Autodesk Fusion 360 part; units mm, degrees
note: some values were not read from the file. Set by a fixed rule: which sketch regions a step uses.
(part 2 of 2)
  line L440 (18.6477, 82.7525) -> (18.6477, 82.7527)
  line L441 (18.6477, 82.7527) -> (18.6477, 82.7525)
  circle A451 centre (18.1478, 85.2926) radius 0.754
  arc A452 (17.648, 85.2925) -> (18.6477, 85.2925) centre (18.1478, 85.2925) ccw
  arc A453 (18.6477, 85.2927) -> (17.648, 85.2927) centre (18.1478, 85.2927) ccw
  line L442 (17.648, 85.2927) -> (17.648, 85.2925)
  line L443 (17.648, 85.2925) -> (17.648, 85.2927)
  line L444 (18.6477, 85.2925) -> (18.6477, 85.2927)
  line L445 (18.6477, 85.2927) -> (18.6477, 85.2925)
  arc A454 (78.2438, 58.2496) -> (78.2438, 59.2496) centre (78.2438, 58.7496) ccw
  arc A455 (78.1938, 59.2496) -> (78.1938, 58.2496) centre (78.1938, 58.7496) ccw
  line L446 (78.2438, 58.2496) -> (78.1938, 58.2496)
  line L447 (78.1938, 58.2496) -> (78.2438, 58.2496)
  line L448 (78.2438, 59.2496) -> (78.1938, 59.2496)
  line L449 (78.1938, 59.2496) -> (78.2438, 59.2496)
  arc A456 (78.2438, 55.7096) -> (78.2438, 56.7096) centre (78.2438, 56.2096) ccw
  arc A457 (78.1938, 56.7096) -> (78.1938, 55.7096) centre (78.1938, 56.2096) ccw
  line L450 (78.2438, 55.7096) -> (78.1938, 55.7096)
  line L451 (78.1938, 55.7096) -> (78.2438, 55.7096)
  line L452 (78.2438, 56.7096) -> (78.1938, 56.7096)
  line L453 (78.1938, 56.7096) -> (78.2438, 56.7096)
  arc A458 (78.2438, 53.1696) -> (78.2438, 54.1696) centre (78.2438, 53.6696) ccw
  arc A459 (78.1938, 54.1696) -> (78.1938, 53.1696) centre (78.1938, 53.6696) ccw
  line L454 (78.2438, 53.1696) -> (78.1938, 53.1696)
  line L455 (78.1938, 53.1696) -> (78.2438, 53.1696)
  line L456 (78.2438, 54.1696) -> (78.1938, 54.1696)
  line L457 (78.1938, 54.1696) -> (78.2438, 54.1696)
  arc A460 (78.2438, 60.7896) -> (78.2438, 61.7896) centre (78.2438, 61.2896) ccw
  arc A461 (78.1938, 61.7896) -> (78.1938, 60.7896) centre (78.1938, 61.2896) ccw
  line L458 (78.2438, 60.7896) -> (78.1938, 60.7896)
  line L459 (78.1938, 60.7896) -> (78.2438, 60.7896)
  line L460 (78.1938, 61.7896) -> (78.2438, 61.7896)
  line L461 (78.2438, 61.7896) -> (78.1938, 61.7896)
  arc A462 (81.4368, 16.5156) -> (81.4368, 17.7156) centre (81.4368, 17.1156) ccw
  arc A463 (83.6368, 17.7156) -> (83.6368, 16.5156) centre (83.6368, 17.1156) ccw
  line L462 (83.6368, 16.5156) -> (81.4368, 16.5156)
  line L463 (81.4368, 16.5156) -> (83.6368, 16.5156)
  line L464 (81.4368, 17.7156) -> (83.6368, 17.7156)
  line L465 (83.6368, 17.7156) -> (81.4368, 17.7156)
  arc A464 (87.6368, 13.0156) -> (86.4368, 13.0156) centre (87.0368, 13.0156) ccw
  arc A465 (86.4368, 15.2156) -> (87.6368, 15.2156) centre (87.0368, 15.2156) ccw
  line L466 (86.4368, 15.2156) -> (86.4368, 13.0156)
  line L467 (86.4368, 13.0156) -> (86.4368, 15.2156)
  line L468 (87.6368, 13.0156) -> (87.6368, 15.2156)
  line L469 (87.6368, 15.2156) -> (87.6368, 13.0156)
  arc A466 (81.4368, 9.9156) -> (81.4368, 11.1156) centre (81.4368, 10.5156) ccw
  arc A467 (83.6368, 11.1156) -> (83.6368, 9.9156) centre (83.6368, 10.5156) ccw
  line L470 (81.4368, 9.9156) -> (83.6368, 9.9156)
  line L471 (83.6368, 9.9156) -> (81.4368, 9.9156)
  line L472 (83.6368, 11.1156) -> (81.4368, 11.1156)
  line L473 (81.4368, 11.1156) -> (83.6368, 11.1156)
  circle A468 centre (83.9338, 61.6706) radius 0.4445
  circle A469 centre (83.9338, 59.1306) radius 0.4445
  circle A470 centre (83.9338, 59.1306) radius 0.7874
  circle A471 centre (83.9338, 56.5906) radius 0.4445
  circle A472 centre (83.9338, 56.5906) radius 0.7874
  circle A473 centre (83.9338, 54.0506) radius 0.4445
  circle A474 centre (83.9338, 54.0506) radius 0.7874
  circle A475 centre (38.3408, 61.2198) radius 1.016
  circle A476 centre (5.3208, 60.9658) radius 1.016
  circle A477 centre (5.3208, 16.0078) radius 1.016
  circle A478 centre (38.3408, 16.0078) radius 1.016
  circle A479 centre (50.5049, 4.6197) radius 1.016
  circle A480 centre (72.4048, 4.6197) radius 1.016
  circle A481 centre (50.5049, 61.1197) radius 1.016
  circle A482 centre (72.4048, 61.1197) radius 1.016
  circle A483 centre (71.3075, 67.3056) radius 1.5
  circle A484 centre (50.9806, 67.3056) radius 1.5
  circle A485 centre (50.9806, 97.8054) radius 1.5
  circle A486 centre (71.3075, 97.8456) radius 1.5
  circle A487 centre (95.8825, 46.7984) radius 1.4999
  circle A488 centre (95.8543, 38.3133) radius 1.4999
  circle A489 centre (19.2908, 71.0686) radius 1
  circle A490 centre (19.2908, 91.8966) radius 1
  circle A491 centre (42.4048, 91.8966) radius 1
  circle A492 centre (42.4048, 71.0686) radius 1
  circle A493 centre (82.5368, 6.5155) radius 1.25
  arc A494 (104.4344, 98.5006) -> (97.6244, 105.3106) centre (97.6244, 98.5006) ccw
  line L474 (3.6444, 105.3106) -> (97.6244, 105.3106)
  arc A495 (3.6444, 105.3106) -> (-3.1656, 98.5006) centre (3.6444, 98.5006) ccw
  line L475 (-3.1656, -5.4794) -> (-3.1656, 98.5006)
  line L476 (104.4344, 98.5006) -> (104.4344, 4.5206)
  line L477 (-3.1656, -5.4794) -> (-3.1656, -49.4794)
  line L478 (104.4344, 4.5206) -> (104.4344, -49.4794)
  line L479 (2.8344, -55.4794) -> (98.4344, -55.4794)
  arc A496 (-3.1656, -49.4794) -> (2.8344, -55.4794) centre (2.8344, -49.4794) ccw
  arc A497 (98.4344, -55.4794) -> (104.4344, -49.4794) centre (98.4344, -49.4794) ccw
  arc A498 (108.4344, 98.5006) -> (97.6244, 109.3106) centre (97.6244, 98.5006) ccw
  line L480 (3.6444, 109.3106) -> (97.6244, 109.3106)
  arc A499 (3.6444, 109.3106) -> (-7.1656, 98.5006) centre (3.6444, 98.5006) ccw
  line L481 (-7.1656, -5.4794) -> (-7.1656, 98.5006)
  line L482 (-7.1656, -5.4794) -> (-7.1656, -49.4794)
  arc A500 (-7.1656, -49.4794) -> (2.8344, -59.4794) centre (2.8344, -49.4794) ccw
  line L483 (2.8344, -59.4794) -> (98.4344, -59.4794)
  arc A501 (98.4344, -59.4794) -> (108.4344, -49.4794) centre (98.4344, -49.4794) ccw
  line L484 (108.4344, 4.5206) -> (108.4344, -49.4794)
  line L485 (108.4344, 98.5006) -> (108.4344, 4.5206)
  arc A502 (105.9344, 98.5006) -> (97.6244, 106.8106) centre (97.6244, 98.5006) ccw
  line L486 (3.6444, 106.8106) -> (97.6244, 106.8106)
  arc A503 (3.6444, 106.8106) -> (-4.6656, 98.5006) centre (3.6444, 98.5006) ccw
  line L487 (-4.6656, -5.4794) -> (-4.6656, 98.5006)
  line L488 (-4.6656, -5.4794) -> (-4.6656, -49.4794)
  arc A504 (-4.6656, -49.4794) -> (2.8344, -56.9794) centre (2.8344, -49.4794) ccw
  line L489 (2.8344, -56.9794) -> (98.4344, -56.9794)
  arc A505 (98.4344, -56.9794) -> (105.9344, -49.4794) centre (98.4344, -49.4794) ccw
  line L490 (105.9344, 4.5206) -> (105.9344, -49.4794)
  line L491 (105.9344, 98.5006) -> (105.9344, 4.5206)
  point P0 (-3.1656, -55.4794)
  point P1 (104.4344, -55.4794)
  dimension "d2" = 50
  dimension "d3" = 60
  dimension "d4" = 6
  dimension "d5" = 6
  dimension "d6" = 56.19
  dimension "d7" = 101.6
  dimension "d8" = -4
  dimension "d13" = 101.6
  dimension "d14" = -1.5
  constraint concentric A0 A494
  constraint concentric A3 A495
  constraint tangent A495 L475
  constraint tangent L474 A495
  constraint tangent A494 L474
  constraint tangent A494 L476
  constraint vertical L477
  constraint parallel L475 L477
  constraint vertical L478
  constraint parallel L476 L478
  constraint perpendicular L478 L479
  constraint coincident P0 L477
  constraint coincident P0 L479
  constraint tangent L477 A496
  constraint tangent L479 A496
  constraint coincident P1 L478
  constraint coincident P1 L479
  constraint tangent L478 A497
  constraint tangent L479 A497
  measures "d2" distance of L475.start P0
  measures "d3" distance of L476.end P1
  measures "d4" radius of A496
  measures "d5" radius of A497
  measures "d6" distance of L57 L479
  measures "d7" distance of L57 L59
  measures "d13" distance of L56.start L58
extrude "Extrude1" add sketch "PCB_wildfire-prediction-system_2026-03-05" along normal blind 3 contours L0 L1 L2 L60 L61 L165 L276 | L0 L1 L2 L32 L90 L122 L275 L276 | L27 L85 L86 L87 | L27 L53 L63 L65 L66 L81 L83 L85 L110 L112 L116 L142 L163 L164 L165 | L32 L33 L83 L90 L165 | L32 L33 L82 L83 L84 L88 L89 L90 L212 | L32 L88 L89 L90 L212 | L23 L60 L61 L101 L104 L121 L142 L163 L165 L173 L268 L270 L273 L274 L276 | L27 L68 L72 L81 L83 L85 L165 | L33 L74 L83 L165 | L32 L88 L122 L124 L179 L181 L189 L195 L212 | L26 L31 L33 L68 L74 L76 L82 L83 L84 L165 L212 | L33 L68 L74 L165 | L1 L61 L261 L276 L281 | L1 L122 L123 L261 L275 L276 L281 | L32 L122 L207 | L32 L122 L124 L182 L189 L198 | L82 L88 L180 L181 L185 L201 L212 | L61 L121 L260 L261 L262 L273 L274 L276 L277 L280 L281 | L53 L112 L142 L163 L173 | L53 L142 L163 | L33 L68 L74 L76 | L25 L26 L27 L68 L72 L165 | L31 L33 L68 L165 | L121 L123 L260 L261 L262 L277 L280 L281 A146 A147 L324 L325 A301 A302 L388 L389 | L9 L16 L91 L124 L182 L189 L190 L194 L197 L198 L202 L203 A111 A112 A113 A266 A267 A268 | L32 L91 L94 L95 L194 L207 | L32 L94 L122 L207 L275 | L16 L124 L140 L179 L180 L181 L183 L184 L185 L186 L187 L188 L189 L190 L191 L192 L193 L195 L196 L200 L201 L204 L205 L206 A113 A268 | L26 L82 L183 L184 L186 L196 L201 L212 | L101 L107 L108 L109 L112 L115 L173 A94 A249 | L53 L112 L163 | L94 L122 L123 L261 L263 L275 L278 L281 | L93 L94 L121 L123 L260 L261 L263 L277 L278 L281 A146 A147 L322 L323 A148 A149 L326 L327 L328 L329 A301 A302 L386 L387 A303 A304 L390 L391 L392 L393 | L32 L94 L207 | L9 L91 L194 L199 L202 A112 A267 | L9 L91 L94 L95 L139 L194 L199 L202 L207 | L26 L137 L141 L212 | L26 L137 L140 L184 L200 L212 | L20 L106 L112 L115 L132 L173 A100 A255 | L53 L112 L173 | L21 L22 L23 L101 L104 L172 L173 | L20 L21 L101 L106 L107 L108 L109 L172 L173 A94 A249 | L53 L110 L112 L113 L114 L132 L133 L144 L163 L164 L173 | L110 L112 L116 L163 L164 | L27 L63 L65 L66 L67 L70 L71 L72 L164 | L25 L26 L27 L49 L67 L71 L72 L78 L79 L165 | L14 L16 L17 L77 L79 L137 L139 L140 L141 L161 L162 L165 L187 L200 | L121 L123 A146 A147 L324 L325 A301 A302 L388 L389 A456 A457 L452 L453 | L121 L123 A146 A147 L322 L323 A301 A302 L386 L387 A456 A457 L450 L451 | L32 L94 L139 L275 | L93 L94 L138 L139 L260 L263 L274 L275 L277 L278 | L32 L94 L139 L207 | L9 L91 A112 A267 A422 | L9 L91 A111 A112 A266 A267 A421 A422 | L16 L124 A113 A268 A423 | L16 L124 A113 A268 A423 | L93 L121 L260 L274 L277 | L93 L121 L268 L274 | L101 L107 A94 A249 A404 | L101 L107 A94 A249 A404 | L46 L47 L49 L50 L78 L79 L96 L97 L164 L165 | L14 L77 L79 L165 | L121 L123 A456 A457 L452 L453 | L121 L123 A456 A457 L450 L451 | L93 L94 L260 L263 L277 L278 L279 A148 L326 L327 A303 L390 L391 | L32 L139 L275 | L32 L138 L139 L274 L275 | L5 L30 L32 L54 L139 L207 L221 L268 L269 L270 L271 L272 L274 L275 | L8 L9 L54 L139 L207 L211 | L9 L91 A422 | L9 L91 A421 A422 | L16 L124 A114 A115 A269 A270 A423 | L16 L124 A114 A115 A269 A270 A423 | L12 L23 L117 L120 L121 L268 L270 A158 A313 | L4 L5 L12 L23 L93 L100 L102 L103 L117 L120 L121 L268 L270 A158 A160 A313 A315 | L93 L138 L268 L274 | L20 L105 L106 L132 L171 L173 A100 A255 | L105 L132 L133 L136 L144 L145 L171 L173 L224 L226 L228 | L101 L107 A93 A248 A404 | L101 L107 A93 A248 A404 | L23 L103 L104 L270 | L5 L22 L23 L24 L103 L104 L221 L270 | L20 L21 L105 L106 L171 L172 L174 | L63 L110 L113 L114 L133 L136 L144 L145 L146 L147 L164 | L14 L77 L96 L161 L165 | L93 L94 A148 A149 L326 L327 L328 L329 A303 A304 L390 L391 L392 L393 A458 A459 L454 L455 L456 L457 | L93 L94 A148 L326 L327 A303 L390 L391 A458 L454 L455 | L260 L263 L279 | L32 L274 L275 | L9 L16 L139 L190 L197 L202 L203 | L8 L9 L16 L17 L139 L211 | L16 L124 A114 A115 A269 A270 A424 A425 | L16 L124 A114 A115 A269 A270 A424 A425 | L16 L139 L140 L187 L188 L190 L191 L192 L193 L204 L205 L206 | L140 L187 L200 | L4 L5 L93 L100 L102 L268 L269 L270 L271 L272 A160 A315 | L30 L32 L138 L268 L274 | L20 L132 A100 A255 A410 | L20 L132 A100 A255 A410 | L101 L107 A93 A248 A403 | L101 L107 A93 A248 A403 | L63 L70 L75 L147 L164 | L40 L45 L49 L67 L78 | L40 L41 L43 L44 L46 L47 L49 L50 L78 L164 | L14 L77 L161 | L96 L97 L130 L164 L165 | L10 L96 L130 L131 L160 L161 L165 L266 L267 | L92 L93 L94 A458 A459 L454 L455 L456 L457 | L92 L93 L94 A458 L454 L455 | L8 L54 L55 L159 L162 L211 | L219 L220 L221 L222 | L16 L124 L125 A424 A425 | L16 L124 L125 A424 A425 | L4 L93 L100 A160 A315 A470 | L4 L93 L100 A160 A315 A470 | L20 L132 A99 A254 A410 | L20 L132 A99 A254 A410 | L133 L136 L144 L145 | L101 L107 A403 | L101 L107 A403 | L5 L103 L270 | L37 L38 L70 L75 L136 L145 L146 L147 L149 L150 L164 L228 | L40 L41 L43 L44 L45 L67 L70 L164 | L14 L15 L17 L161 L162 | L14 L19 L77 L161 | L18 L19 L77 L96 L161 | L10 L18 L96 L160 L161 A25 A180 | L130 L164 L165 L166 | L8 L17 L162 L211 | L12 L117 A158 A313 A468 | L12 L117 A158 A313 A468 | L4 L93 L100 A159 A314 A470 | L4 L93 L100 A159 A314 A470 | L20 L132 A99 A254 A409 | L20 L132 A99 A254 A409 | L105 L226 L257 L259 | L105 L226 L258 L259 | L35 L37 L150 L164 | L7 L8 L15 L17 L18 L19 L96 L98 L162 A27 A182 | L97 L130 L164 L178 | L50 L51 L97 L164 L177 L178 | L7 L8 L10 L18 L55 L96 L98 L159 L160 L162 A25 A27 A180 A182 | L55 L159 L160 | L12 L117 A468 | L12 L117 A468 | L4 L93 L100 A159 A314 A469 | L4 L93 L100 A159 A314 A469 | L20 L132 A409 | L20 L132 A409 | L105 L136 L224 L228 L253 L257 L259 | L39 L105 L223 L225 L227 L231 L232 L239 L240 L242 L251 L252 L253 L258 L259 | L34 L35 L37 L38 L149 L150 | L37 L38 L149 L150 | L35 L43 L150 L153 L154 L164 | L42 L97 L175 L176 L177 L178 | L51 L97 L177 L178 | L42 L43 L50 L51 L152 L153 L164 L177 | L10 L18 A25 A180 A335 | L10 L18 A25 A180 A335 | L10 L55 L160 L266 | L10 L11 L131 L266 L267 A156 L342 L343 L344 L345 A311 L406 L407 L408 L409 A466 L470 L471 L472 L473 | L10 L11 L131 L264 L265 L266 L267 A157 L342 L343 L344 L345 A312 L406 L407 L408 L409 A467 L470 L471 L472 L473 | L4 L93 L100 A469 | L4 L93 L100 A469 | L38 L136 L228 L253 L254 | L39 L105 L135 L136 L253 | L39 L105 L251 L252 L253 | L34 L35 L148 L149 L150 L151 | L42 L51 L97 L177 | L10 L18 A335 | L10 L18 A335 | L7 L98 A27 A182 A337 | L7 L98 A27 A182 A337 | L131 A156 L342 L343 A311 L406 L407 L470 L471 | L131 A157 L342 L343 A312 L406 L407 L470 L471 | L38 L39 L135 L136 L253 L254 | L34 L38 L228 L254 | L34 L38 L149 L228 | L39 L105 L252 | L36 L39 L105 L135 L252 | L42 L43 L150 L152 L153 L154 | L42 L43 L152 L153 | L7 L98 A26 A181 A337 | L7 L98 A26 A181 A337 | L11 L131 A156 A311 A466 L470 L471 L472 L473 | L118 L131 A157 A312 A467 L470 L471 | L34 L36 L38 L39 L135 L254 | L34 L135 L225 L228 L229 L235 L243 L244 L252 L254 | L36 L39 L105 L234 L236 L238 L242 L252 L255 | L36 L105 L252 L255 | L225 L229 L230 L231 L232 L233 L234 L235 L236 L237 L238 L239 L240 L241 L242 L243 L244 L245 L246 L247 L248 L249 L250 | L7 L98 A26 A181 A336 | L7 L98 A26 A181 A336 | L11 A157 L344 L345 A312 L408 L409 L472 L473 | L11 A156 L344 L345 A311 L408 L409 L472 L473 | L11 L118 A157 A312 A467 L472 L473 | A156 A311 A466 L470 L471 | A157 A312 A467 L470 L471 | L34 L36 L135 L252 L254 | L36 L135 L252 | L36 L105 L135 L229 L230 L237 L241 L252 L255 | L225 L249 L250 | L6 L7 L98 A336 | L6 L7 L98 A336 | L118 A157 A312 A467 | L118 A157 A312 A467 | A156 A311 A466 | L36 L105 L233 L237 L238 L255 | L151 L155 L156 L158 | A157 A312 A467 L472 L473 | A156 A311 A466 L472 L473 | L225 L245 L246 | L225 L247 L248 | L13 L24 A126 A281 A436 | L13 L24 A126 A281 A436 | L13 L24 A125 A280 A436 | L13 L24 A125 A280 A436 | L13 L24 A125 A280 A435 | L13 L24 A125 A280 A435 | L13 L24 A435 | L13 L24 A435 | L55 A152 L336 L337 A307 L400 L401 L464 L465 | A152 A153 A307 A308 A462 A463 L462 L463 L464 L465 | L55 A153 L336 L337 A308 L400 L401 L464 L465 | A152 A307 A462 L464 L465 | A153 A308 A463 L464 L465 | A152 A307 A462 | A153 A308 A463 | A152 A307 A462 L462 L463 | A153 A308 A463 L462 L463 | A152 A153 L334 L335 A307 A308 L398 L399 L462 L463 | L56 L57 L58 L59 A0 A1 A2 A3 | L119 A155 L338 L339 A310 L402 L403 L466 L467 | L119 A154 L338 L339 A309 L402 L403 L466 L467 | A154 A155 A309 A310 L466 L467 L468 L469 | A155 A310 A465 L466 L467 L468 L469 | A154 A309 A464 L466 L467 L468 L469 | A154 A155 L340 L341 A309 A310 L404 L405 L468 L469 | L128 L129 A415 | L128 L129 A415 | L128 L129 A105 A260 A415 | L128 L129 A105 A260 A415 | L128 L129 A105 A260 A416 | L128 L129 A105 A260 A416 | L128 L129 A106 A261 A416 | L128 L129 A106 A261 A416 | L167 L168 L169 L170 | A6 | A7 | A8 | A9 | A10 A165 | A11 A166 | A12 A167 | A13 A168 | A14 A169 | A15 A170 | A16 A171 | A17 A172 | A18 A173 | A19 A174 | A20 A175 | A21 A176 | A22 A177 | A23 A178 | A24 A179 | A28 A183 | A29 A184 | A30 A185 | A31 A186 | A32 A187 | A33 A188 | A34 A189 | A35 A190 | A36 A191 | A37 A192 | A38 A193 | A39 A194 | A40 A195 | A41 A196 | A42 A197 | A43 A198 | A44 A199 | A45 A200 | A46 A201 | A47 A202 | A48 A203 | A49 A204 | A50 A205 | A51 A206 | A52 A207 | A53 A208 | A54 A209 | A55 A210 | A56 A211 | A57 A212 | A58 A213 | A59 A214 | A60 A215 | A61 A216 | A62 A217 | A63 A218 | A64 A219 | A65 A220 | A66 A221 | A67 A222 | A68 A223 | A69 A224 | A70 A225 | A71 A226 | A72 A227 | A73 A228 | A74 A229 | A75 A230 | A76 A231 | A77 A232 | A78 A233 | A79 A234 | A80 A235 | A81 A236 | A82 A237 | A83 A238 | A84 A239 | A85 A240 | A86 A241 | A87 A242 | A88 A243 | A89 A244 | A90 A245 | A91 A246 | A92 A247 | A95 A250 | A96 A251 | A97 A252 | A98 A253 | A101 A256 | A102 A257 | A103 A258 | A104 A259 | A107 A262 | A108 A263 | A109 A264 | A110 A265 | A116 A271 | A117 A118 A272 A273 | A119 A274 | A120 A121 A275 A276 | A122 A277 | A123 A124 A278 A279 | A127 A282 | A128 A283 | A129 A284 | A130 A285 | A131 A286 | A132 A287 | A133 A134 A288 A289 | A135 A290 | A136 A137 A291 A292 | A138 A293 | A139 A140 A294 A295 | A141 A296 | A142 A143 A297 A298 | A144 A145 L318 L319 L320 L321 A299 A300 L382 L383 L384 L385 | A150 A151 L330 L331 L332 L333 A305 A306 L394 L395 L396 L397 | A161 A316 | A162 A317 | A163 A318 | A164 A319 | A320 | A321 | A322 | A323 | A324 | A325 | A326 | A327 | A328 | A329 | A330 | A331 | A332 | A333 | A334 | A338 | A339 | A340 | A341 | A342 | A343 | A344 | A345 | A346 | A347 | A348 | A349 | A350 | A351 | A352 | A353 | A354 | A355 | A356 | A357 | A358 | A359 | A360 | A361 | A362 | A363 | A364 | A365 | A366 | A367 | A368 | A369 | A370 | A371 | A372 | A373 | A374 | A375 | A376 | A377 | A378 | A379 | A380 | A381 | A382 | A383 | A384 | A385 | A386 | A387 | A388 | A389 | A390 | A391 | A392 | A393 | A394 | A395 | A396 | A397 | A398 | A399 | A400 | A401 | A402 | A405 | A406 | A407 | A408 | A411 | A412 | A413 | A414 | A417 | A418 | A419 | A420 | A426 | A427 A428 | A429 | A430 A431 | A432 | A433 A434 | A437 | A438 | A439 | A440 | A441 | A442 | A443 A444 | A445 | A446 A447 | A448 | A449 A450 | A451 | A452 A453 | A454 A455 L446 L447 L448 L449 | A460 A461 L458 L459 L460 L461 | A471 | A472 | A473 | A474 | A475 | A476 | A477 | A478 | A479 | A480 | A481 | A482 | A483 | A484 | A485 | A486 | A487 | A488 | A489 | A490 | A491 | A492 | A493 | A494 L474 A495 L475 L476 L477 L478 L479 A496 A497 makes body 1
extrude "Extrude2" add sketch "PCB_wildfire-prediction-system_2026-03-05" along normal blind 2 separate body contours A498 L480 A499 L481 L482 A500 L483 A501 L484 L485 | A502 L486 A503 L487 L488 A504 L489 A505 L490 L491 makes body 2
extrude "Extrude3" add sketch "PCB_wildfire-prediction-system_2026-03-05" along normal blind 30 separate body contours A498 L480 A499 L481 L482 A500 L483 A501 L484 L485 makes body 3
sketch "Mics and power" plane through (-7.1656, 0, 0) normal (-1, 0, 0) x (0, -1, 0)
  line L0 (-98.5006, 0) -> (49.4794, 0)
  line L1 (49.4794, 0) -> (49.4794, 30)
  line L2 (49.4794, 30) -> (-98.5006, 30)
  line L3 (-98.5006, 30) -> (-98.5006, 0)
  line L4 (-84.4519, 20.5) -> (-60.4519, 20.5)
  line L5 (-60.4519, 20.5) -> (-60.4519, 3.5)
  line L6 (-60.4519, 3.5) -> (-84.4519, 3.5)
  line L7 (-84.4519, 3.5) -> (-84.4519, 20.5)
  line L8 (33.4794, 12.5) -> (45.4794, 12.5)
  line L9 (45.4794, 12.5) -> (45.4794, 3.5)
  line L10 (45.4794, 3.5) -> (33.4794, 3.5)
  line L11 (33.4794, 3.5) -> (33.4794, 12.5)
  line L12 (13, 14.5) -> (22, 14.5)
  line L13 (22, 14.5) -> (22, 3.5)
  line L14 (22, 3.5) -> (13, 3.5)
  line L15 (13, 3.5) -> (13, 14.5)
  dimension "d17" = 24
  dimension "d18" = 17
  dimension "d29" = 12
  dimension "d30" = 9
  dimension "d31" = 4
  dimension "d32" = 17.5
  dimension "d35" = 9
  dimension "d36" = 11
  dimension "d38" = 3.5
  dimension "d41" = 3.5
  constraint horizontal L4
  constraint vertical L5
  constraint horizontal L6
  constraint vertical L7
  constraint horizontal L8
  constraint vertical L9
  constraint horizontal L10
  constraint vertical L11
  constraint horizontal L12
  constraint vertical L13
  constraint horizontal L14
  constraint vertical L15
  measures "d17" distance of L4.start L4.end
  measures "d18" distance of L4.start L6.end
  measures "d29" distance of L8.start L8.end
  measures "d30" distance of L8.start L10.end
  measures "d31" distance of L1 L9
  measures "d32" distance of L2 L8
  measures "d35" distance of L12.start L12.end
  measures "d36" distance of L12.start L14.end
  measures "d38" distance of L0 L14
  measures "d41" distance of L0 L6
extrude "Extrude4" cut sketch "Mics and power" against normal blind 5 contours L4 L5 L6 L7 bodies 1 2 3
sketch "PM2" plane through (108.4344, 0, 0) normal (1, 0, 0) x (0, 1, 0)
  line L0 (-49.4794, 0) -> (98.5006, 0)
  line L1 (98.5006, 0) -> (98.5006, 30)
  line L2 (98.5006, 30) -> (-49.4794, 30)
  line L3 (-49.4794, 30) -> (-49.4794, 0)
  line L4 (-40.0146, 2.6533) -> (0.9854, 2.6533)
  line L5 (0.9854, 2.6533) -> (0.9854, 19.6533)
  line L6 (0.9854, 19.6533) -> (-40.0146, 19.6533)
  line L7 (-40.0146, 19.6533) -> (-40.0146, 2.6533)
  circle A0 centre (20, 10) radius 2.5
  dimension "d21" = 41
  dimension "d22" = 17
  dimension "d25" = 5
  constraint horizontal L4
  constraint vertical L5
  constraint horizontal L6
  constraint vertical L7
  measures "d21" distance of L4.start L4.end
  measures "d22" distance of L4.start L6.end
  measures "d25" diameter of A0
extrude "Extrude5" cut sketch "PM2" against normal blind 5 contours L4 L5 L6 L7 bodies 1 3
extrude "Extrude6" cut sketch "PM2" against normal blind 5 contours A0 bodies 3
extrude "Extrude7" cut sketch "Mics and power" against normal blind 4 contours L8 L9 L10 L11 bodies 3
extrude "Extrude8" cut sketch "Mics and power" against normal blind 10 contours L12 L13 L14 L15 bodies 3
sketch "Sketch4" plane through (0, 0, 30) normal (0, 0, 1) x (-1, 0, 0)
  arc A0 (-3.6444, -106.8106) -> (4.6656, -98.5006) centre (-3.6444, -98.5006) ccw
  line L0 (-3.6444, -106.8106) -> (-97.6244, -106.8106)
  arc A1 (-105.9344, -98.5006) -> (-97.6244, -106.8106) centre (-97.6244, -98.5006) ccw
  line L1 (-105.9344, -98.5006) -> (-105.9344, 49.4794)
  arc A2 (-98.4344, 56.9794) -> (-105.9344, 49.4794) centre (-98.4344, 49.4794) ccw
  line L2 (-98.4344, 56.9794) -> (-2.8344, 56.9794)
  arc A3 (4.6656, 49.4794) -> (-2.8344, 56.9794) centre (-2.8344, 49.4794) ccw
  line L3 (4.6656, 49.4794) -> (4.6656, -98.5006)
  arc A4 (-3.6444, -109.3106) -> (7.1656, -98.5006) centre (-3.6444, -98.5006) ccw
  line L4 (7.1656, -98.5006) -> (7.1656, 49.4794)
  arc A5 (7.1656, 49.4794) -> (-2.8344, 59.4794) centre (-2.8344, 49.4794) ccw
  line L5 (-2.8344, 59.4794) -> (-98.4344, 59.4794)
  arc A6 (-98.4344, 59.4794) -> (-108.4344, 49.4794) centre (-98.4344, 49.4794) ccw
  line L6 (-108.4344, 49.4794) -> (-108.4344, -98.5006)
  arc A7 (-108.4344, -98.5006) -> (-97.6244, -109.3106) centre (-97.6244, -98.5006) ccw
  line L7 (-97.6244, -109.3106) -> (-3.6444, -109.3106)
extrude "Extrude9" add sketch "Sketch4" along normal blind 3 separate body contours A0 L0 A1 L1 A2 L2 A3 L3 | A4 L4 A5 L5 A6 L6 A7 L7 makes body 4
sketch "Sketch5" plane through (0, 0, 33) normal (0, 0, 1) x (-1, 0, 0)
  line L0 (-97.6244, -109.3106) -> (-3.6444, -109.3106)
  arc A0 (-3.6444, -109.3106) -> (7.1656, -98.5006) centre (-3.6444, -98.5006) ccw
  line L1 (7.1656, -98.5006) -> (7.1656, 49.4794)
  arc A1 (7.1656, 49.4794) -> (-2.8344, 59.4794) centre (-2.8344, 49.4794) ccw
  line L2 (-2.8344, 59.4794) -> (-98.4344, 59.4794)
  arc A2 (-98.4344, 59.4794) -> (-108.4344, 49.4794) centre (-98.4344, 49.4794) ccw
  line L3 (-108.4344, 49.4794) -> (-108.4344, -98.5006)
  arc A3 (-108.4344, -98.5006) -> (-97.6244, -109.3106) centre (-97.6244, -98.5006) ccw
  circle A4 centre (-82.1061, -83.0443) radius 7.5
  line L4 (5.1656, -98.5006) -> (5.1656, 49.4794)
  arc A5 (5.1656, 49.4794) -> (-2.8344, 57.4794) centre (-2.8344, 49.4794) ccw
  line L5 (-2.8344, 57.4794) -> (-98.4344, 57.4794)
  arc A6 (-98.4344, 57.4794) -> (-106.4344, 49.4794) centre (-98.4344, 49.4794) ccw
  line L6 (-106.4344, 49.4794) -> (-106.4344, -98.5006)
  arc A7 (-106.4344, -98.5006) -> (-97.6244, -107.3106) centre (-97.6244, -98.5006) ccw
  line L7 (-97.6244, -107.3106) -> (-3.6444, -107.3106)
  arc A8 (-3.6444, -107.3106) -> (5.1656, -98.5006) centre (-3.6444, -98.5006) ccw
  dimension "d44" = 15
  dimension "d47" = -2
  measures "d44" diameter of A4
extrude "Extrude10" cut sketch "Sketch5" against normal blind 10 contours A4 bodies 4
extrude "Extrude11" add sketch "Sketch5" against normal blind 4.5 contours L4 A5 L5 A6 L6 A7 L7 A8 bodies 4
fillet "Fillet1" radius 0.5 16 edges at (-7.1656, 84.4519, 12) (-7.1656, 72.4519, 20.5) (-7.1656, 72.4519, 3.5) (-7.1656, 60.4519, 12) (-7.1656, -13, 9) (-7.1656, -17.5, 14.5) (-7.1656, -22, 9) (-7.1656, -17.5, 3.5) (-7.1656, -33.4794, 8) (-7.1656, -39.4794, 12.5) (-7.1656, -39.4794, 3.5) (-7.1656, -45.4794, 8) (108.4344, -40.0146, 11.1533) (108.4344, -19.5146, 19.6533) (108.4344, 0.9854, 11.1533) (108.4344, -19.5146, 2.6533) on bodies 3
